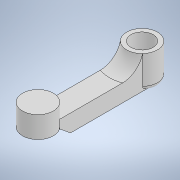
# Autodesk Inventor part: Рулевая тяга правая
Saved by Autodesk Inventor 2020 (Build 240168000, 168)
## iProperties
Created: 2021-08-11
Part Number: Рулевая тяга правая
Material: Типовые
Document SubType Name: Modeling
Designer: Антон
Density: 1 g/cm^3
Appearance: По умолчанию
Author: Антон
Autodesk Inventor part; units mm, degrees
ref_plane "YZ Plane" through (0, 0, 0) normal (1, 0, 0) x (0, 1, 0)
ref_plane "XZ Plane" through (0, 0, 0) normal (0, 1, 0) x (-1, 0, 0)
ref_plane "XY Plane" through (0, 0, 0) normal (0, 0, 1) x (1, 0, 0)
sketch "Эскиз6" plane through (0, 0, 0) normal (0, 1, 0) x (-1, 0, 0)
  circle A0 centre (0, 0) radius 2.575
  circle A1 centre (0, 0) radius 3.575
  dimension "d11" = 5.15
  dimension "d12" = 1
  constraints: 2 centre point, 2 coincident
  measures "d11" diameter of A0
  measures "d12" radial gap between concentric circles of A1 A0
extrude "Выдавливание5" add sketch "Эскиз6" along normal blind 4
ref_plane "РабПлоскость1" through (0, 1.6, 0) normal (0, -1, 0) x (1, 0, 0)
sketch "Эскиз1" plane through (0, 1.6, 0) normal (0, 1, 0) x (-1, 0, 0)
  circle A0 centre (0, 0) radius 2.575 projected
  line L0 (-2.575, 0) -> (2.575, 0)
  line L1 (2.575, 0) -> (2.575, -24.1495)
  line L2 (2.575, -24.1495) -> (-2.575, -24.1495)
  line L3 (-2.575, -24.1495) -> (-2.575, 0)
  circle A1 centre (0, -24.1495) radius 3.575
  circle A2 centre (0, 0) radius 3.575 projected
  point P0 (2.575, -2.4799)
  point P1 (-2.575, -2.4799)
  point P2 (-2.575, -21.6696)
  point P3 (2.575, -21.6696)
  dimension "d15" = 24.1495
  constraints: 8 end point, 2 midpoint, 2 parallel, 1 centre point, 1 coincident, 1 equal radius, 1 horizontal, 1 perpendicular, 1 tangent
  measures "d15" distance of L2.end L0.start
extrude "Выдавливание1" add sketch "Эскиз1" against normal blind 4 separate body contours L1 A1 L3 A2 | A1 L3 L2 L1 | L1 L2 L3 A1
chamfer "Фаска1" distance 2 angle 45 1 edges at (0, -2.4, -3.575)
sketch "Эскиз7" plane through (0, 1.6, 0) normal (0, -1, 0) x (1, 0, 0)
  arc A0 (-2.575, -21.6696) -> (2.575, -21.6696) centre (0, -24.1495) ccw projected
  circle A1 centre (0, -24.1495) radius 3.575
  point P0 (0, 0)
  point P1 (-2.575, -21.6696)
  constraints: 1 coincident, 3 other
extrude "Выдавливание6" add sketch "Эскиз7" against normal blind 3.6 bodies 2
sketch "Эскиз8" plane through (0, 5.2, -24.1495) normal (0, 1, 0) x (-1, 0, 0)
  circle A0 centre (0, 0) radius 3.575 projected
  circle A1 centre (0, 0) radius 2.575
  circle A2 centre (0, 24.1495) radius 2.575 projected
  constraints: 1 centre point, 1 coincident, 1 equal radius
extrude "Выдавливание7" cut sketch "Эскиз8" against normal blind 4 contours A1 bodies 2
fillet "Сопряжение1" radius 4 1 edges at (0, 1.6, -20.5745)
fillet "Сопряжение2" radius 1 1 edges at (0, -2.4, -27.7245)
sketch "Эскиз9" plane through (0, 4, 0) normal (0, 1, 0) x (1, 0, 0)
  circle A0 centre (0, 0) radius 3.575 projected
extrude "Выдавливание8" add sketch "Эскиз9" along normal blind 1 bodies 1
